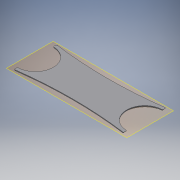
# Autodesk Inventor part: cap
Saved by Autodesk Inventor 2017 (Build 210142000, 142)
## iProperties
Created: 2017-06-23
Part Number: cap
Material: Generic
Document SubType Name: Modeling
Designer: erwin
Density: 1 g/cm^3
Appearance: Default
Author: erwin
Autodesk Inventor part; units mm, degrees
ref_plane "YZ Plane" through (0, 0, 0) normal (1, 0, 0) x (0, 1, 0)
ref_plane "XZ Plane" through (0, 0, 0) normal (0, 1, 0) x (-1, 0, 0)
ref_plane "XY Plane" through (0, 0, 0) normal (0, 0, 1) x (1, 0, 0)
ref_plane "Work Plane1" through (0, 0, 0) normal (0, 0, 1) x (1, 0, 0)
sketch "Sketch1" plane through (0, 0, 0) normal (0, 0, 1) x (1, 0, 0)
  arc A0 (-60.8058, -23.1869) -> (-60.8058, 23.1869) centre (-67, 0) ccw projected
  arc A1 (-60.8058, 23.1869) -> (60.8058, 23.1869) centre (0, 521.4907) ccw projected
  arc A2 (60.8058, 23.1869) -> (60.8058, -23.1869) centre (67, 0) ccw projected
  arc A3 (60.8058, -23.1869) -> (-60.8058, -23.1869) centre (0, -521.4907) ccw projected
  arc A4 (-67, -22) -> (-67, 22) centre (-67, 0) ccw projected
  line L0 (-67, -26) -> (-67, -22) projected
  arc A5 (67, -26) -> (-67, -26) centre (0, -521.4907) ccw projected
  line L1 (67, -22) -> (67, -26) projected
  arc A6 (67, 22) -> (67, -22) centre (67, 0) ccw projected
  line L2 (67, 26) -> (67, 22) projected
  arc A7 (-67, 26) -> (67, 26) centre (0, 521.4907) ccw projected
  line L3 (-67, 22) -> (-67, 26) projected
  point P0 (0, 0)
extrude "Extrusion1" add sketch "Sketch1" along normal blind 1 contours A0 A1 A2 A3 | A4 L3 A7 L2 A6 L1 A5 L0
fillet "Fillet1" radius 1 12 edges at (67, -26, 0.5) (67, -22, 0.5) (67, -24, 0) (67, 22, 0.5) (67, 26, 0.5) (67, 24, 0) (-67, -26, 0.5) (-67, -22, 0.5) (-67, -24, 0) (-67, 22, 0.5) (-67, 26, 0.5) (-67, 24, 0)
sketch "Sketch2" plane through (0, 0, 0) normal (0, 0, -1) x (-1, 0, 0)
  arc A0 (-60.8058, -23.1869) -> (-60.8058, 23.1869) centre (-67, 0) ccw projected
  arc A1 (60.8058, -23.1869) -> (-60.8058, -23.1869) centre (0, -521.4907) ccw projected
  arc A2 (-60.8058, 23.1869) -> (60.8058, 23.1869) centre (0, 521.4907) ccw projected
  arc A3 (60.8058, 23.1869) -> (60.8058, -23.1869) centre (67, 0) ccw projected
  arc A4 (-59.6234, 22.9433) -> (59.6234, 22.9433) centre (0, 521.4907) ccw
  arc A5 (-59.6234, -22.9433) -> (-59.6234, 22.9433) centre (-67, 0) ccw
  arc A6 (59.6234, -22.9433) -> (-59.6234, -22.9433) centre (0, -521.4907) ccw
  arc A7 (59.6234, 22.9433) -> (59.6234, -22.9433) centre (67, 0) ccw
  arc A8 (-53.6579, 21.2603) -> (53.6579, 21.2603) centre (0, 521.4907) ccw
  arc A9 (-53.6579, -21.2603) -> (-53.6579, 21.2603) centre (-67, 0) ccw
  arc A10 (53.6579, -21.2603) -> (-53.6579, -21.2603) centre (0, -521.4907) ccw
  arc A11 (53.6579, 21.2603) -> (53.6579, -21.2603) centre (67, 0) ccw
  point P0 (0, 0)
  dimension "d3" = 0.1
  dimension "d4" = 1
  constraints: 16 point on circle, 8 centre point, 6 other
  measures "d3" radial gap between concentric circles of A2 A4
  measures "d4" radial gap between concentric circles of A4 A8
extrude "Extrusion2" add sketch "Sketch2" along normal blind 2 contours A4 A7 A6 A5
sketch "Sketch3" plane through (0, 0, 1) normal (0, 0, 1) x (1, 0, 0)
  circle A0 centre (2, 0) radius 6
  line L0 (-19.7, -8.9844) -> (0.5, -8.9844)
  line L1 (0.5, -8.9844) -> (0.5, -15.4844)
  line L2 (0.5, -15.4844) -> (-19.7, -15.4844)
  line L3 (-19.7, -15.4844) -> (-19.7, -8.9844)
  line L4 (-19.95, -15.7344) -> (0.75, -15.7344)
  line L5 (0.75, -15.7344) -> (0.75, -8.7344)
  line L6 (0.75, -8.7344) -> (-19.95, -8.7344)
  line L7 (-19.95, -8.7344) -> (-19.95, -15.7344)
  circle A1 centre (2, 0) radius 6.25
  line L8 (1.75, -16.7344) -> (-20.95, -16.7344)
  line L9 (-20.95, -16.7344) -> (-20.95, -7.7344)
  line L10 (-20.95, -7.7344) -> (1.75, -7.7344)
  line L11 (1.75, -7.7344) -> (1.75, -16.7344)
  point P0 (0, 0)
  dimension "d7" = 0.25
  dimension "d8" = 0.25
  dimension "d11" = 1
  constraints: 24 end point, 2 centre point, 6 other
  measures "d7" distance between parallel lines of L2 L4
  measures "d8" radial gap between concentric circles of A0 A1
  measures "d11" distance between parallel lines of L4 L8
extrude "Extrusion3" cut sketch "Sketch3" against normal blind 1 contours A0 | L0 L1 L2 L3 | L7 L6 L5 L4 | A1 | L8 L9 L10 L11
body "Solid1"
